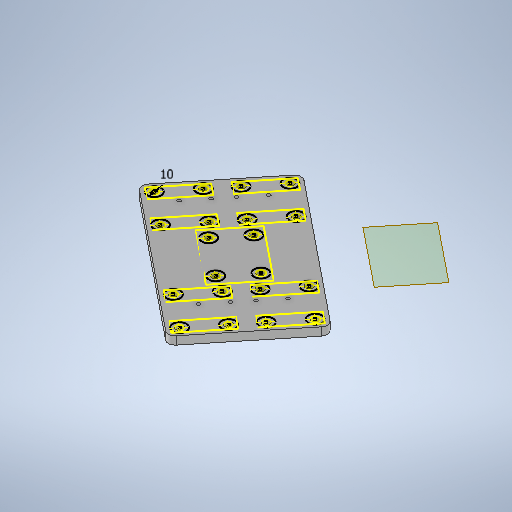
# Autodesk Inventor part: X_PLATE_V2
Saved by Autodesk Inventor 2025.2 (Build 292293000, 293)
## iProperties
Created: 2026-02-06
Part Number: X_PLATE_V2
Material: Generic
Document SubType Name: Modeling
Designer: composite
Density: 1 g/cm^3
Appearance: Default
Author: composite
Autodesk Inventor part; units mm, degrees
ref_plane "YZ Plane" through (0, 0, 0) normal (1, 0, 0) x (0, 1, 0)
ref_plane "XZ Plane" through (0, 0, 0) normal (0, 1, 0) x (-1, 0, 0)
ref_plane "XY Plane" through (0, 0, 0) normal (0, 0, 1) x (1, 0, 0)
ref_plane "Work Plane1" through (45.5839, 2165.7463, -107.1675) normal (0, -1, 0) x (0.6267496, 0, -0.7792208)
sketch "Sketch1" plane through (45.5839, 2165.7463, -107.1675) normal (0, -1, 0) x (0.6267496, 0, -0.7792208)
  line L0 (-112.4658, 32.3282) -> (-112.4521, 21.5782) projected
  line L1 (-112.4521, 21.5782) -> (-77.2521, 21.6232) projected
  line L2 (-77.2521, 21.6232) -> (-77.2659, 32.3732) projected
  line L3 (-112.4658, 32.3282) -> (-77.2659, 32.3732) projected
  circle A0 centre (-81.8604, 28.1173) radius 2.5 projected
  circle A1 centre (-107.8604, 28.084) radius 2.5 projected
  line L4 (-66.4659, 32.387) -> (-66.4521, 21.637) projected
  line L5 (-66.4521, 21.637) -> (-31.2521, 21.682) projected
  line L6 (-31.2521, 21.682) -> (-31.2659, 32.432) projected
  line L7 (-66.4659, 32.387) -> (-31.2659, 32.432) projected
  circle A2 centre (-35.8605, 28.1761) radius 2.5 projected
  circle A3 centre (-61.8604, 28.1429) radius 2.5 projected
  line L8 (-31.0953, -100.9679) -> (-31.109, -90.2179) projected
  line L9 (-31.109, -90.2179) -> (-66.309, -90.2629) projected
  line L10 (-66.309, -90.2629) -> (-66.2953, -101.0129) projected
  line L11 (-31.0953, -100.9679) -> (-66.2953, -101.0129) projected
  circle A4 centre (-61.7007, -96.757) radius 2.5 projected
  circle A5 centre (-35.7007, -96.7238) radius 2.5 projected
  line L12 (-77.0953, -101.0267) -> (-77.109, -90.2767) projected
  line L13 (-77.109, -90.2767) -> (-112.309, -90.3217) projected
  line L14 (-112.309, -90.3217) -> (-112.2952, -101.0717) projected
  line L15 (-77.0953, -101.0267) -> (-112.2952, -101.0717) projected
  circle A6 centre (-107.7007, -96.8159) radius 2.5 projected
  circle A7 centre (-81.7007, -96.7826) radius 2.5 projected
  line L16 (-77.1314, -72.7767) -> (-77.1451, -62.0268) projected
  line L17 (-77.1451, -62.0268) -> (-112.3451, -62.0718) projected
  line L18 (-112.3451, -62.0718) -> (-112.3314, -72.8218) projected
  line L19 (-112.3314, -72.8218) -> (-77.1314, -72.7767) projected
  circle A8 centre (-107.7397, -66.3159) radius 2.5 projected
  circle A9 centre (-81.7397, -66.2826) radius 2.5 projected
  line L20 (-31.1314, -72.7179) -> (-31.1452, -61.9679) projected
  line L21 (-31.1452, -61.9679) -> (-66.3451, -62.0129) projected
  line L22 (-66.3451, -62.0129) -> (-66.3314, -72.7629) projected
  line L23 (-66.3314, -72.7629) -> (-31.1314, -72.7179) projected
  circle A10 centre (-61.7397, -66.2571) radius 2.5 projected
  circle A11 centre (-35.7397, -66.2238) radius 2.5 projected
  circle A12 centre (-83.7582, -51.8352) radius 2.5 projected
  circle A13 centre (-59.803, -16.8045) radius 2.5 projected
  circle A14 centre (-59.7582, -51.8045) radius 2.5 projected
  circle A15 centre (-83.8029, -16.8352) radius 2.5 projected
  line L24 (-89.8125, -9.3429) -> (-89.7486, -59.3429) projected
  line L25 (-89.7486, -59.3429) -> (-53.7486, -59.2968) projected
  line L26 (-53.8125, -9.2969) -> (-53.7486, -59.2968) projected
  line L27 (-89.8125, -9.3429) -> (-53.8125, -9.2969) projected
  line L28 (-66.4297, 4.137) -> (-66.416, -6.613) projected
  line L29 (-66.416, -6.613) -> (-31.216, -6.568) projected
  line L30 (-31.216, -6.568) -> (-31.2298, 4.182) projected
  line L31 (-31.2298, 4.182) -> (-66.4297, 4.137) projected
  circle A16 centre (-35.8214, -2.3239) radius 2.5 projected
  circle A17 centre (-61.8214, -2.3571) radius 2.5 projected
  line L32 (-112.4297, 4.0782) -> (-112.416, -6.6718) projected
  line L33 (-112.416, -6.6718) -> (-77.216, -6.6268) projected
  line L34 (-77.216, -6.6268) -> (-77.2297, 4.1232) projected
  line L35 (-77.2297, 4.1232) -> (-112.4297, 4.0782) projected
  circle A18 centre (-81.8214, -2.3827) radius 2.5 projected
  circle A19 centre (-107.8214, -2.4159) radius 2.5 projected
  point P0 (-112.0768, 31.6472)
sketch "Sketch2" plane through (45.5839, 2165.7463, -107.1675) normal (0, -1, 0) x (0.6267496, 0, -0.7792208)
  circle A0 centre (-35.7007, -96.7238) radius 2.5 projected
  line L0 (-112.2952, -101.0717) -> (-31.0953, -100.9679)
  line L1 (-31.0953, -100.9679) -> (-31.2659, 32.432)
  line L2 (-31.2659, 32.432) -> (-112.4658, 32.3282)
  line L3 (-112.4658, 32.3282) -> (-112.2952, -101.0717)
  circle A1 centre (-107.7007, -96.8159) radius 2.75
  circle A2 centre (-81.7007, -96.7826) radius 2.75
  circle A3 centre (-61.7007, -96.757) radius 2.75
  circle A4 centre (-35.7007, -96.7238) radius 2.75
  circle A5 centre (-35.7397, -66.2238) radius 2.75
  circle A6 centre (-61.7397, -66.2571) radius 2.75
  circle A7 centre (-81.7397, -66.2826) radius 2.75
  circle A8 centre (-107.7397, -66.3159) radius 2.75
  circle A9 centre (-83.7582, -51.8352) radius 2.75
  circle A10 centre (-59.7582, -51.8045) radius 2.75
  circle A11 centre (-59.803, -16.8045) radius 2.75
  circle A12 centre (-83.8029, -16.8352) radius 2.75
  circle A13 centre (-107.8214, -2.4159) radius 2.75
  circle A14 centre (-81.8214, -2.3827) radius 2.75
  circle A15 centre (-61.8214, -2.3571) radius 2.75
  circle A16 centre (-35.8214, -2.3239) radius 2.75
  circle A17 centre (-35.8605, 28.1761) radius 2.75
  circle A18 centre (-61.8604, 28.1429) radius 2.75
  circle A19 centre (-81.8604, 28.1173) radius 2.75
  circle A20 centre (-107.8604, 28.084) radius 2.75
  line L4 (-28.0915, -103.9641) -> (-115.2914, -104.0756)
  line L5 (-115.2914, -104.0756) -> (-115.4697, 35.3243)
  line L6 (-115.4697, 35.3243) -> (-28.2697, 35.4358)
  line L7 (-28.2697, 35.4358) -> (-28.0915, -103.9641)
  point P0 (-112.0768, 31.6472)
  dimension "d0" = 5.5
  dimension "d1" = 5.5
  dimension "d2" = 5.5
  dimension "d3" = 5.5
  dimension "d4" = 5.5
  dimension "d5" = 5.5
  dimension "d6" = 5.5
  dimension "d7" = 5.5
  dimension "d8" = 5.5
  dimension "d9" = 5.5
  dimension "d10" = 5.5
  dimension "d11" = 5.5
  dimension "d12" = 5.5
  dimension "d13" = 5.5
  dimension "d14" = 5.5
  dimension "d15" = 5.5
  dimension "d16" = 5.5
  dimension "d17" = 5.5
  dimension "d18" = 5.5
  dimension "d19" = 5.5
  dimension "d42" = 3
  constraints: 21 coincident, 20 centre point, 16 end point, 4 parallel, 2 perpendicular, 3 other
  measures "d0" diameter of A1
  measures "d1" diameter of A2
  measures "d2" diameter of A3
  measures "d3" diameter of A4
  measures "d4" diameter of A5
  measures "d5" diameter of A6
  measures "d6" diameter of A7
  measures "d7" diameter of A8
  measures "d8" diameter of A9
  measures "d9" diameter of A10
  measures "d10" diameter of A11
  measures "d11" diameter of A12
  measures "d12" diameter of A13
  measures "d13" diameter of A14
  measures "d14" diameter of A15
  measures "d15" diameter of A16
  measures "d16" diameter of A17
  measures "d17" diameter of A18
  measures "d18" diameter of A19
  measures "d19" diameter of A20
  measures "d42" distance between parallel lines of L0 L4
extrude "Extrusion1" add sketch "Sketch2" along normal blind 6 contours L3 L2 L1 L0 | L4 L5 L6 L7
sketch "Sketch3" plane through (45.5839, 2159.7463, -107.1675) normal (0, -1, 0) x (0.7792208, 0, 0.6267496)
  circle A0 centre (-87.2395, 47.9629) radius 1.25
  circle A1 centre (-87.2612, 64.9629) radius 1.25
  circle A2 centre (-87.2785, 78.4628) radius 1.25
  circle A3 centre (-87.3002, 95.4628) radius 1.25
  circle A4 centre (7.7605, 48.0844) radius 1.25
  circle A5 centre (7.7387, 65.0843) radius 1.25
  circle A6 centre (7.7215, 78.5843) radius 1.25
  circle A7 centre (7.6997, 95.5843) radius 1.25
  line L0 (-87.2395, 47.9629) -> (-87.2141, 28.1129) construction
  line L1 (-87.3002, 95.4628) -> (-87.3256, 115.3128) construction
  line L2 (-90.2767, 77.109) -> (-90.3217, 112.309) projected
  line L3 (7.7605, 48.0844) -> (7.7387, 65.0843) construction
  line L4 (7.7387, 65.0843) -> (7.7215, 78.5843) construction
  line L5 (7.7215, 78.5843) -> (7.6997, 95.5843) construction
  line L6 (-87.2395, 47.9629) -> (-87.2612, 64.9629) construction
  line L7 (-87.2612, 64.9629) -> (-87.2785, 78.4628) construction
  line L8 (-87.2785, 78.4628) -> (-87.3002, 95.4628) construction
  line L9 (-87.2395, 47.9629) -> (7.7605, 48.0844) construction
  line L10 (7.7387, 65.0843) -> (-87.2612, 64.9629) construction
  line L11 (-87.2785, 78.4628) -> (7.7215, 78.5843) construction
  line L12 (7.6997, 95.5843) -> (-87.3002, 95.4628) construction
  line L13 (35.3243, 115.4697) -> (-104.0756, 115.2914) projected
  line L14 (-104.0756, 115.2914) -> (-103.9641, 28.0915) projected
  line L15 (-103.9641, 28.0915) -> (35.4358, 28.2697) projected
  line L16 (35.4358, 28.2697) -> (35.3243, 115.4697) projected
  point P0 (31.6472, 112.0768)
  dimension "d26" = 2.5
  dimension "d30" = 17
  dimension "d31" = 13.5
  dimension "d32" = 17
  dimension "d33" = 95
  dimension "d43" = 3
  constraints: 24 end point, 8 centre point, 7 equal radius, 6 parallel, 4 collinear, 3 equal length, 2 perpendicular, 2 point on line
  measures "d26" diameter of A4
  measures "d30" distance of L0.start L6.end
  measures "d31" distance of L7.end L6.end
  measures "d32" distance of L1.start L7.end
  measures "d33" distance of L3.start L0.start
  measures "d43" distance between parallel lines of L2 L1
extrude "Extrusion2" cut sketch "Sketch3" against normal blind 10 contours A0 | A1 | A2 | A3 | A4 | A5 | A6 | A7
sketch "Sketch4" plane through (45.5839, 2165.7463, -107.1675) normal (0, 1, 0) x (0.7792208, 0, 0.6267496)
  circle A0 centre (-2.4159, -107.8214) radius 2.5 projected
  circle A1 centre (-96.8159, -107.7007) radius 2.75 projected
  circle A2 centre (-96.8159, -107.7007) radius 5
  circle A3 centre (-96.7826, -81.7007) radius 2.75 projected
  circle A4 centre (-96.7826, -81.7007) radius 5
  circle A5 centre (-96.757, -61.7007) radius 5
  circle A6 centre (-96.7238, -35.7007) radius 5
  circle A7 centre (-66.2238, -35.7397) radius 5
  circle A8 centre (-66.2571, -61.7397) radius 5
  circle A9 centre (-66.2826, -81.7397) radius 5
  circle A10 centre (-66.3159, -107.7397) radius 5
  circle A11 centre (-51.8352, -83.7582) radius 2.75 projected
  circle A12 centre (-51.8352, -83.7582) radius 5
  circle A13 centre (-51.8045, -59.7582) radius 2.75 projected
  circle A14 centre (-51.8045, -59.7582) radius 5
  circle A15 centre (-16.8045, -59.803) radius 2.75 projected
  circle A16 centre (-16.8045, -59.803) radius 5
  circle A17 centre (-16.8352, -83.8029) radius 5
  circle A18 centre (-2.4159, -107.8214) radius 5
  circle A19 centre (-2.3827, -81.8214) radius 2.75 projected
  circle A20 centre (-2.3827, -81.8214) radius 5
  circle A21 centre (-2.3571, -61.8214) radius 5
  circle A22 centre (-2.3239, -35.8214) radius 5
  circle A23 centre (28.084, -107.8604) radius 5
  circle A24 centre (28.1173, -81.8604) radius 5
  circle A25 centre (28.1429, -61.8604) radius 5
  circle A26 centre (28.1761, -35.8605) radius 2.75 projected
  circle A27 centre (28.1761, -35.8605) radius 5
  point P0 (31.6472, -112.0768)
  point P1 (-51.8352, -83.7582)
  dimension "d39" = 10
  constraints: 20 centre point, 20 coincident, 19 equal radius
  measures "d39" diameter of A2
fillet "Fillet1" radius 5 4 edges at (-107.7728, 2162.7463, -82.5594) (-53.0333, 2162.7463, -150.4375) (0.7388, 2162.7463, 4.9484) (55.4782, 2162.7463, -62.9297)
sketch "Sketch5" plane through (45.5839, 2159.7463, -107.1675) normal (0, -1, 0) x (0.7792208, 0, 0.6267496)
  circle A0 centre (-96.7238, 35.7007) radius 5 projected
  circle A1 centre (-96.757, 61.7007) radius 5 projected
  circle A2 centre (-96.7826, 81.7007) radius 5 projected
  circle A3 centre (-96.8159, 107.7007) radius 5 projected
  circle A4 centre (-66.3159, 107.7397) radius 5 projected
  circle A5 centre (-66.2826, 81.7397) radius 5 projected
  circle A6 centre (-66.2571, 61.7397) radius 5 projected
  circle A7 centre (-66.2238, 35.7397) radius 5 projected
  circle A8 centre (-51.8045, 59.7582) radius 5 projected
  circle A9 centre (-51.8352, 83.7582) radius 5 projected
  circle A10 centre (-16.8352, 83.8029) radius 5 projected
  circle A11 centre (-16.8045, 59.803) radius 5 projected
  circle A12 centre (-2.4159, 107.8214) radius 5 projected
  circle A13 centre (-2.3827, 81.8214) radius 5 projected
  circle A14 centre (-2.3571, 61.8214) radius 5 projected
  circle A15 centre (-2.3239, 35.8214) radius 5 projected
  circle A16 centre (28.1761, 35.8605) radius 5 projected
  circle A17 centre (28.1429, 61.8604) radius 5 projected
  circle A18 centre (28.1173, 81.8604) radius 5 projected
  circle A19 centre (28.084, 107.8604) radius 5 projected
  point P0 (31.6472, 112.0768)
extrude "Extrusion4" cut sketch "Sketch5" against normal blind 3
body "Solid1"
